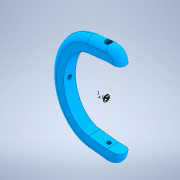
# Autodesk Inventor part: BodyDampener V2
Saved by Autodesk Inventor 2022.2 (Build 262287030, 287C)
## iProperties
Created: 2022-03-24
Part Number: BodyDampener V2
Material: Generic
Document SubType Name: Modeling
Designer: Jochen
Density: 1 g/cm^3
Appearance: Default
Author: Jochen
Autodesk Inventor part; units mm, degrees
ref_plane "YZ Plane" through (0, 0, 0) normal (1, 0, 0) x (0, 1, 0)
ref_plane "XZ Plane" through (0, 0, 0) normal (0, 1, 0) x (-1, 0, 0)
ref_plane "XY Plane" through (0, 0, 0) normal (0, 0, 1) x (1, 0, 0)
sketch "Sketch1" plane through (0, 0, 0) normal (0, 0, 1) x (1, 0, 0)
  line L0 (0, 28.4285) -> (0, -28.4285) construction
  line L1 (0, 28.4285) -> (-43.231, 28.4285) construction
  line L2 (-43.231, -28.4285) -> (-43.231, 28.4285) construction
  line L3 (0, -28.4285) -> (-43.231, -28.4285) construction
  line L4 (-28, -28.4285) -> (-28, 28.4285) construction
  line L5 (0, 28.4285) -> (-28, 28.4285) construction
  line L6 (0, 28.4285) -> (-9, 27.4285)
  ellipse E0 centre (-7.2715, 0) end of major axis (-7.2715, -27.5244) minor radius 20.7285 (-9, 27.4285) -> (-9, -27.4285) ccw
  line L7 (0, 28.4285) -> (0, -28.4285) construction
  line L8 (0, 28.4285) -> (0, -28.4285)
  line L9 (0, -28.4285) -> (-28, -28.4285) construction
  line L10 (0, -28.4285) -> (-28, -28.4285)
  line L11 (0, -28.4285) -> (-28, -28.4285)
  line L12 (0, -28.4285) -> (-9, -27.4285)
  line L13 (0, 0.1054) -> (0, 0.565) construction
  line L14 (0, -28.4285) -> (18, -30.4285) construction
  line L15 (18, -30.4285) -> (18, -28.4285) construction
  line L16 (-43.231, 28.4285) -> (-43.231, -28.4285) construction
  line L17 (-43.231, 0) -> (0, 0) construction
  line L18 (0, -28.4285) -> (0, 28.4285) construction
  line L19 (-9, -27.4285) -> (-9, 27.4285) construction
  line L20 (0, -60.9505) -> (0, 75.8697) construction
  line L21 (-75.6, 0) -> (33.6, 0) construction
  line L22 (-10.1043, 37.3673) -> (3.8957, 38.9229)
  line L23 (3.8957, -38.9229) -> (-10.1043, -37.3673)
  line L24 (0, 28.4285) -> (5, 28.9841)
  line L25 (0, -28.4285) -> (10, -29.5396)
  line L26 (5, 28.9841) -> (15, 28.9841)
  line L27 (5, -28.9841) -> (15, -28.9841)
  arc A0 (15, 28.9841) -> (3.8957, 38.9229) centre (5, 28.9841) ccw
  arc A1 (3.8957, -38.9229) -> (15, -28.9841) centre (5, -28.9841) ccw
  line L28 (10, -28.9841) -> (10, -29.5396)
  line L29 (-9, 27.4285) -> (-10.1043, 37.3673) construction
  spline S0 degree 5 poles (-10.1043, -37.3674) (-10.8216, -37.2877) (-11.536, -37.1829) (-12.2466, -37.0531) (-16.6054, -36.0996) (-20.7313, -34.2288) (-23.8743, -32.0866) (-29.4463, -26.9126) (-33.4267, -20.4278) (-35.0135, -16.9404) (-37.409, -9.6142) (-38.2, -1.9459) (-38.2, 1.9459) (-37.409, 9.6142) (-35.0135, 16.9404) (-33.4267, 20.4278) (-29.4463, 26.9126) (-23.8743, 32.0866) (-20.7313, 34.2288) (-16.6054, 36.0996) (-12.2466, 37.0531) (-11.536, 37.1829) (-10.8216, 37.2877) (-10.1043, 37.3674) knots 0 0 0 0 0 0 0.035408 0.035408 0.035408 0.21878 0.21878 0.21878 0.405168 0.405168 0.405168 0.594832 0.594832 0.594832 0.78122 0.78122 0.78122 0.964592 0.964592 0.964592 1 1 1 1 1 1
  point P0 (-60, 28.4445)
  point P1 (-13, 43)
  point P2 (-13, 56.324)
  point P3 (-13, 11)
  point P4 (-13, 0.565)
  point P5 (0, 0.3352)
  point P6 (-9, 0)
  dimension "d7" = 10
  dimension "d0" = 2
  dimension "d1" = 18
  dimension "d2" = 28
  dimension "d3" = 9
  dimension "d4" = 19
  dimension "d5" = 56.857
  dimension "d8" = 5
  dimension "d9" = 10
  constraints: 57 end point, 7 midpoint, 4 perpendicular, 4 point on circle, 4 point on line, 3 vertical, 2 centre point, 2 collinear, 2 horizontal, 2 line through centre, 2 parallel, 2 tangent, 1 coincident, 1 vertical alignment, 12 other
  measures "d0" distance of L14.end L15.end
  measures "d1" distance from line of L0.end L15
  measures "d2" distance between parallel lines of L0 L4
  measures "d3" distance between parallel lines of L0 L19
  measures "d4" distance between parallel lines of L19 L4
  measures "d5" distance of L2.start L1.end
  measures "d8" distance from line of L0 L24.end
  measures "d9" distance of L24.end L26.end
extrude "Extrusion1" add sketch "Sketch1" along normal blind 9 contours L6 E0 L12 L10 S0 L22 A0 L26 L24 | L25 L28 L27 A1 L23 S0 L10 | L27 L28 L25
fillet "Fillet1" radius 4.5 10 edges at (-3.1043, -38.1451, 9) (11.6692, -36.4353, 9) (-3.1043, 38.1451, 9) (11.6692, 36.4353, 9) (-38, 0, 9) (-3.1043, -38.1451, 0) (11.6692, -36.4353, 0) (-3.1043, 38.1451, 0) (11.6692, 36.4353, 0) (-38, 0, 0)
sketch "Sketch2" plane through (0, 0, 0) normal (0, 1, 0) x (-1, 0, 0)
  line L0 (0, -1.8) -> (0, 10.8) construction
  line L1 (1.6, 0) -> (-6.1, 0) construction
  circle A0 centre (-2, 4.5) radius 1.5
  line L2 (-5, 0) -> (-5, 9) projected
  circle A1 centre (-2, 4.5) radius 2.5
  point P0 (0, 0)
  dimension "d13" = 3
  dimension "d14" = 3
  dimension "d15" = 4.5
  dimension "d18" = 5
  constraints: 2 centre point, 1 coincident
  measures "d13" diameter of A0
  measures "d14" distance from line of A0.centre L2
  measures "d15" distance from line of L1 A0.centre
  measures "d18" diameter of A1
extrude "Extrusion3" add sketch "Sketch2" along normal through all both and the other way through all separate body contours A0 | A1
extrude "Extrusion4" cut sketch "Sketch2" along normal mid plane 70 contours A0 | A1 bodies 2
combine bodies "Combine1" operation type subtract main body 1 bodies to subtract 2
extrude "Extrusion2" cut sketch "Sketch2" along normal through all both and the other way through all contours A0 bodies 1
sketch "Sketch3" plane through (0, 0, 0) normal (1, 0, 0) x (0, 1, 0)
  line L0 (37.3673, 4.5) -> (-37.3673, 4.5) construction
  circle A0 centre (0, 4.5) radius 1.5
  circle A1 centre (0, 4.5) radius 2.25
  point P0 (0, 0)
  dimension "d23" = 3
  dimension "d24" = 4.5
  constraints: 2 centre point, 1 coincident, 1 midpoint
  measures "d23" diameter of A0
  measures "d24" diameter of A1
extrude "Extrusion6" add sketch "Sketch3" against normal blind 40 separate body contours A0
extrude "Extrusion7" add sketch "Sketch3" along normal blind 5 from surface at -40 contours A0 | A1 bodies 3
combine bodies "Combine2" operation type subtract main body 1 bodies to subtract 3
